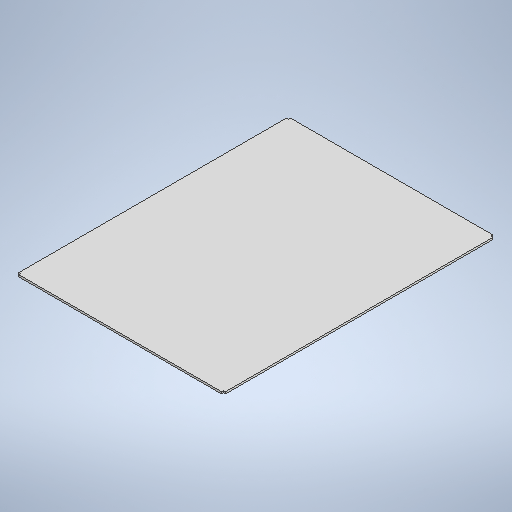
# Autodesk Inventor part: Podloga
Saved by Autodesk Inventor 2026.2 (Build 302298010, 298A)
## iProperties
Created: 2026-04-29
Part Number: Podloga
Material: Ogólny
Document SubType Name: Modeling
Designer: Patryk
Density: 1 g/cm^3
Appearance: Domyślna
Author: Patryk
Autodesk Inventor part; units mm, degrees
ref_plane "YZ Plane" through (0, 0, 0) normal (1, 0, 0) x (0, 1, 0)
ref_plane "XZ Plane" through (0, 0, 0) normal (0, 1, 0) x (-1, 0, 0)
ref_plane "XY Plane" through (0, 0, 0) normal (0, 0, 1) x (1, 0, 0)
sketch "Szkic1" plane through (0, 0, 0) normal (0, 1, 0) x (-1, 0, 0)
  line L0 (-159, -209) -> (159, -209)
  line L1 (159, -209) -> (159, 209)
  line L2 (159, 209) -> (-159, 209)
  line L3 (-159, 209) -> (-159, -209)
  line L4 (-159, -209) -> (159, 209) construction
  line L5 (159, -209) -> (-159, 209) construction
  line L6 (159, 209) -> (156, 209)
  line L7 (156, 209) -> (156, 206)
  line L8 (156, 206) -> (159, 206)
  line L9 (159, 206) -> (159, 209)
  line L10 (-159, 209) -> (-156, 209)
  line L11 (-156, 209) -> (-156, 206)
  line L12 (-156, 206) -> (-159, 206)
  line L13 (-159, 206) -> (-159, 209)
  line L14 (-159, -209) -> (-156, -209)
  line L15 (-156, -209) -> (-156, -206)
  line L16 (-156, -206) -> (-159, -206)
  line L17 (-159, -206) -> (-159, -209)
  line L18 (159, -209) -> (156, -209)
  line L19 (156, -209) -> (156, -206)
  line L20 (156, -206) -> (159, -206)
  line L21 (159, -206) -> (159, -209)
  point P0 (0, 0)
  dimension "d0" = 318
  dimension "d1" = 418
  dimension "d2" = 3
  dimension "d3" = 3
  dimension "d4" = 3
  dimension "d5" = 3
  dimension "d6" = 3
  dimension "d7" = 3
  dimension "d8" = 3
  dimension "d9" = 3
  constraints: 44 end point, 10 parallel, 5 horizontal, 5 perpendicular, 2 midpoint
  measures "d0" distance of L2.end L1.end
  measures "d1" distance of L1.end L0.end
  measures "d2" distance of L8.end L7.end
  measures "d3" distance of L7.end L6.end
  measures "d4" distance of L11.end L12.end
  measures "d5" distance of L10.end L11.end
  measures "d6" distance of L16.end L15.end
  measures "d7" distance of L15.end L14.end
  measures "d8" distance of L19.end L20.end
  measures "d9" distance of L18.end L19.end
extrude "Wyciągnięcie proste1" add sketch "Szkic1" along normal mid plane 3 contours L15 L16 L3 L12 L11 L2 L7 L8 L1 L20 L19 L0
